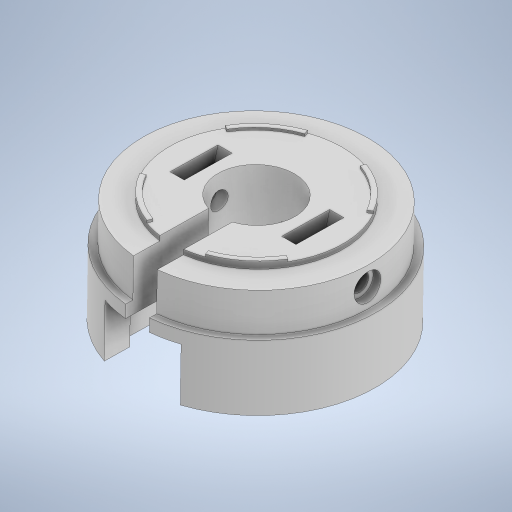
# Autodesk Inventor part: PiezoMount
Saved by Autodesk Inventor 2023 (Build 270158000, 158)
## iProperties
Created: 2023-02-27
Part Number: PiezoMount
Material: Generic
Document SubType Name: Modeling
Designer: maste
Density: 1 g/cm^3
Appearance: Default
Author: maste
Autodesk Inventor part; units mm, degrees
ref_plane "YZ Plane" through (0, 0, 0) normal (1, 0, 0) x (0, 1, 0)
ref_plane "XY Plane" through (0, 0, 0) normal (0, 0, 1) x (1, 0, 0)
sketch "Sketch1" plane through (0, 0, 0) normal (0, 0, 1) x (1, 0, 0)
  circle A0 centre (0, 0) radius 25
  dimension "d2" = 50
  constraints: 1 centre point, 1 coincident
  measures "d2" diameter of A0
extrude "piezo surface" add sketch "Sketch1" along normal blind 8
sketch "Sketch4" plane through (0, 0, 0) normal (0, 0, -1) x (-1, 0, 0)
  circle A0 centre (0, 0) radius 25 projected
extrude "Depth extension to surface" add sketch "Sketch4" along normal blind 3.62
sketch "Sketch2" plane through (0, 0, 8) normal (0, 0, 1) x (1, 0, 0)
  circle A0 centre (0, 0) radius 17.95
  circle A1 centre (0, 0) radius 18.75
  line L0 (0, 0) -> (18.75, 0)
  arc A2 (18.75, 0) -> (16.238, 9.375) centre (0, 0) ccw
  line L1 (0, 0) -> (16.238, 9.375) construction
  line L2 (0, 0) -> (18.75, 0) construction
  line L3 (16.238, 9.375) -> (15.5452, 8.975)
  line L4 (0, 0) -> (0, 18.75)
  line L5 (0, 0) -> (0, -18.75)
  line L6 (0, 0) -> (-18.75, 0)
  line L7 (0, 0) -> (-16.238, -9.375)
  line L8 (0, 0) -> (-9.375, 16.238)
  line L9 (0, 0) -> (9.375, -16.238)
  point P0 (17.95, 0)
  point P1 (8.975, -15.5452)
  point P2 (0, -17.95)
  point P3 (-15.5452, -8.975)
  point P4 (-17.95, 0)
  point P5 (-8.975, 15.5452)
  point P6 (0, 17.95)
  dimension "d3" = 35.9
  dimension "d4" = 37.5
  dimension "d5" = 30
  constraints: 20 end point, 4 point on line, 3 coincident, 2 perpendicular, 2 point on circle, 1 centre point, 1 horizontal, 1 vertical, 12 other
  measures "d5" angle of L2 L1
sketch "Sketch3" plane through (0, 0, 8) normal (0, 0, 1) x (1, 0, 0)
  line L0 (0, 0) -> (8.975, -15.5452)
  arc A0 (17.95, 0) -> (15.5452, 8.975) centre (0, 0) ccw projected
  line L1 (0, 0) -> (17.95, 0)
  arc A1 (0, -17.95) -> (8.975, -15.5452) centre (0, 0) ccw projected
  line L2 (8.975, -15.5452) -> (17.95, 0)
  line L3 (13.4625, -7.7726) -> (0, 0)
  line L4 (13.4625, -7.7726) -> (4.8022, -2.7726)
  line L5 (13.4625, -7.7726) -> (4.8022, -2.7726)
  line L6 (13.4625, -7.7726) -> (4.8022, -2.7726)
  line L7 (4.8022, -2.7726) -> (6.0522, -0.6075)
  line L8 (6.0522, -0.6075) -> (14.7125, -5.6075)
  line L9 (14.7125, -5.6075) -> (13.4625, -7.7726)
  line L10 (13.4625, -7.7726) -> (4.8022, -2.7726)
  line L11 (4.8022, -2.7726) -> (3.5522, -4.9376)
  line L12 (3.5522, -4.9376) -> (12.2125, -9.9376)
  line L13 (12.2125, -9.9376) -> (13.4625, -7.7726)
  line L14 (12.2125, -9.9376) -> (14.7125, -5.6075)
  line L15 (14.7125, -5.6075) -> (16.4446, -6.6075)
  line L16 (16.4446, -6.6075) -> (13.9446, -10.9376)
  line L17 (13.9446, -10.9376) -> (12.2125, -9.9376)
  line L18 (-4.802, 2.7724) -> (-3.552, 4.9375)
  line L19 (-3.552, 4.9375) -> (-13.9443, 10.9375)
  line L20 (-4.802, 2.7724) -> (-6.052, 0.6074)
  line L21 (-6.052, 0.6074) -> (-16.4443, 6.6074)
  line L22 (-16.4443, 6.6074) -> (-23.8055, 10.8574)
  line L23 (-23.8055, 10.8574) -> (-21.3055, 15.1875)
  line L24 (-21.3055, 15.1875) -> (-13.9443, 10.9375)
  line L25 (-5.5448, 2.5) -> (-17.5448, 2.5)
  line L26 (-5.5448, 0) -> (-5.5448, 2.5)
  line L27 (-5.5448, 0) -> (-5.5448, -2.5)
  line L28 (-5.5448, -2.5) -> (-17.5448, -2.5)
  line L29 (-17.5448, -2.5) -> (-26.0448, -2.5)
  line L30 (-26.0448, -2.5) -> (-26.0448, 2.5)
  line L31 (-26.0448, 2.5) -> (-17.5448, 2.5)
  point P0 (14.7125, -5.6075)
  point P1 (12.2125, -9.9376)
  point P2 (12.2125, -9.9376)
  dimension "d37" = 10
  dimension "d38" = 2.5
  dimension "d39" = 2.5
  dimension "d40" = 2
  dimension "d49" = 10
  dimension "d69" = 30
  dimension "d71" = 20.5
  dimension "d72" = 5
  constraints: 64 end point, 7 parallel, 4 collinear, 3 perpendicular, 1 midpoint, 1 point on line, 15 other
  measures "d37" distance of L3.start L4.end
  measures "d38" distance of L4.end L7.end
  measures "d39" distance of L11.end L4.end
  measures "d40" distance of L8.end L15.end
  measures "d49" distance between parallel lines of L11 L13
  measures "d71" distance between parallel lines of L30 L27
  measures "d72" distance between parallel lines of L25 L28
extrude "Microphone Wire Hole" cut sketch "Sketch3" against normal blind 14 contours L26 L27 L28 L29 L30 L31 L25 L21 L20 | L20 L21 L25 L26
sketch "Sketch5" plane through (0, 0, -3.62) normal (0, 0, -1) x (-1, 0, 0)
  line L0 (16, -16) -> (-16, -16)
  line L1 (-16, -16) -> (-16, 16)
  line L2 (-16, 16) -> (16, 16)
  line L3 (16, 16) -> (16, -16)
  line L4 (16, -16) -> (-16, 16) construction
  line L5 (-16, -16) -> (16, 16) construction
  circle A0 centre (0, 0) radius 20
  point P0 (-12, -16)
  point P1 (12, -16)
  point P2 (-16, 12)
  point P3 (-16, -12)
  point P4 (16, 12)
  point P5 (16, -12)
  point P6 (12, 16)
  point P7 (-12, 16)
  dimension "d18" = 32
  dimension "d19" = 32
  dimension "d54" = 40
  constraints: 12 end point, 2 midpoint, 2 parallel, 1 centre point, 1 coincident, 1 horizontal, 1 perpendicular
  measures "d18" distance of L0.start L0.end
  measures "d19" distance of L0.end L1.end
  measures "d54" diameter of A0
extrude "Circuit chamber" cut sketch "Sketch5" against normal blind 3
sketch "Sketch6" plane through (-16, -16, -3.62) normal (1, 0, 0) x (0, 0, -1)
  line L0 (0, 4) -> (0, 0) projected
  line L1 (0, 32) -> (-3, 32) projected
  line L2 (-3, 32) -> (-3, 28) projected
  line L3 (0, 0) -> (-3, 0) projected
  line L4 (-3, 4) -> (-3, 0) projected
  line L5 (0, 32) -> (0, 28) projected
  line L6 (0, 4) -> (-3, 4) projected
  line L7 (0, 18.5) -> (0, 13.5) projected
  line L8 (-11.62, 13.5) -> (-11.62, 18.5) projected
  line L9 (-3, 32) -> (-3, 28) projected
  line L10 (-3, 32) -> (-3, 32) projected
  line L11 (-3, 28) -> (-3, 32) projected
  line L12 (-3, 4) -> (-3, 28) projected
  line L13 (-3, 0) -> (-3, 4) projected
  line L14 (-3, 0) -> (-3, 0) projected
  line L15 (-3, 4) -> (-3, 0) projected
  line L16 (-3, 13.5) -> (-3, 4) projected
  line L17 (0, 18.5) -> (0, 13.5) projected
  line L18 (0, 13.5) -> (0, 4) projected
  line L19 (0, 4) -> (0, 0) projected
  line L20 (0, 0) -> (0, 0) projected
  line L21 (0, 0) -> (0, 4) projected
  line L22 (0, 4) -> (0, 28) projected
  line L23 (0, 28) -> (0, 32) projected
  line L24 (0, 32) -> (0, 32) projected
  line L25 (0, 32) -> (0, 28) projected
  line L26 (-11.62, 16) -> (0, 16)
  line L27 (0, 16) -> (-3, 16)
  line L28 (-3, 16) -> (-3, 24)
  line L29 (-3, 24) -> (0, 24)
  line L30 (0, 24) -> (0, 16)
  line L31 (0, 16) -> (-3, 16)
  line L32 (-3, 16) -> (-3, 8)
  line L33 (-3, 8) -> (0, 8)
  line L34 (0, 8) -> (0, 16)
  line L35 (0, 28) -> (0, 18.5) projected
  line L36 (-3, 18.5) -> (-3, 13.5) projected
  line L37 (-3, 28) -> (-3, 18.5) projected
  line L38 (0, 28) -> (-3, 28) projected
  line L39 (0, 18.5) -> (-11.62, 18.5) projected
  line L40 (-11.62, 13.5) -> (0, 13.5) projected
  point P0 (0, -9)
  point P1 (0, 41)
  point P2 (-11, 41)
  point P3 (-11, -9)
  point P4 (0, -9)
  point P5 (0, 41)
  point P6 (-3, 4)
  point P7 (-3, 8)
  point P8 (0, 8)
  point P9 (-3, 16)
  point P10 (-3, 13.5)
  point P11 (0, 13.5)
  point P12 (0, 18.5)
  dimension "d65" = 8
  dimension "d66" = 8
  constraints: 18 end point, 4 parallel, 2 horizontal, 2 midpoint, 2 perpendicular, 2 point on line
  measures "d65" distance of L27.end L28.end
  measures "d66" distance of L32.end L31.end
extrude "port vent" cut sketch "Sketch6" against normal blind 30 contours L33 L12 L40 L18 | L39 L12 L29 L22
sketch "Sketch7" plane through (0, 0, -3.62) normal (0, 0, -1) x (-1, 0, 0)
  line L0 (0, 0) -> (0, -17.5)
  line L1 (0, 0) -> (0, 17.5)
  dimension "d25" = 17.5
  dimension "d26" = 17.5
  constraints: 4 end point, 2 coincident, 2 vertical
  measures "d25" distance of L0.start L0.end
  measures "d26" distance of L0.start L1.end
hole "screw holes" at (0, 17.5, -3.62) at (0, -17.5, -3.62) direction (0, 0, 1) diameter 3.7 depth 4 tip angle 118
sketch "Sketch8" plane through (0, 0, -3.62) normal (0, 0, -1) x (-1, 0, 0)
  circle A0 centre (0, 0) radius 22.75
  line L0 (21.4137, 11) -> (22.4499, 11) projected
  line L1 (22.4499, 11) -> (19.9139, 11)
  arc A1 (23.6854, 8) -> (23.6854, -8) centre (0, 0) ccw projected
  line L2 (24.6779, -4) -> (22.3956, -4)
  arc A2 (24.8747, 2.5) -> (24.8747, -2.5) centre (0, 0) ccw projected
  arc A3 (-16, 12) -> (-16, -12) centre (0, 0) ccw projected
  arc A4 (-12, -16) -> (12, -16) centre (0, 0) ccw projected
  point P0 (12.5, 7.5)
  point P1 (15.0629, 9)
  point P2 (19.2094, 16)
  point P3 (19.2094, -16)
  point P4 (19.9139, 11)
  point P5 (16.7033, 11)
  point P6 (24.6779, 4)
  point P7 (21.9317, -12)
  dimension "d34" = 45.5
  constraints: 4 end point, 2 point on circle, 1 centre point, 1 coincident, 1 horizontal, 1 parallel, 1 other
  measures "d34" diameter of A0
sketch "Sketch10" plane through (0, 0, -3.62) normal (0, 0, -1) x (-1, 0, 0)
  arc A0 (23.6854, 8) -> (23.6854, -8) centre (0, 0) ccw projected
  arc A1 (16, -12) -> (18.3303, -8) centre (0, 0) ccw projected
  line L0 (16, -16) -> (12, -16) projected
  arc A2 (-12, -16) -> (12, -16) centre (0, 0) ccw projected
  line L1 (-12, -16) -> (-16, -16) projected
  line L2 (-16, -16) -> (-16, -12) projected
  arc A3 (-16, 12) -> (-16, -12) centre (0, 0) ccw projected
  line L3 (-16, 12) -> (-16, 16) projected
  line L4 (-16, 16) -> (-12, 16) projected
  arc A4 (12, 16) -> (-12, 16) centre (0, 0) ccw projected
  line L5 (12, 16) -> (16, 16) projected
  line L6 (16, 16) -> (16, 12) projected
  line L7 (18.3303, 8) -> (23.6854, 8) projected
  line L8 (23.6854, -8) -> (18.3303, -8) projected
  line L9 (16, -12) -> (16, -16) projected
  arc A5 (18.3303, 8) -> (16, 12) centre (0, 0) ccw projected
extrude "Base Extension" add sketch "Sketch10" along normal blind 10
sketch "Sketch13" plane through (0, 0, 8) normal (0, 0, 1) x (0, 1, 0)
  circle A0 centre (0, 0) radius 25
  circle A1 centre (0, 0) radius 23.5
  dimension "d55" = 47
  dimension "d59" = 50
  constraints: 2 centre point, 2 coincident
  measures "d55" diameter of A1
  measures "d59" diameter of A0
extrude "Rim for flush with diaphragm lock" cut sketch "Sketch13" against normal blind 8
sketch "Sketch14" plane through (-16, 12.1244, -3) normal (1, 0, 0) x (0, 0, -1)
  line L0 (10.62, -4.1244) -> (10.62, -20.1244) projected
  line L1 (-3, 11.3756) -> (-11, 11.3756) projected
  line L2 (-11, 11.3756) -> (-11, -35.6244) projected
  line L3 (-3, -9.6244) -> (-3, -14.6244) projected
  line L4 (-2.38, -20.1244) -> (10.62, -20.1244) projected
  line L5 (10.62, -4.1244) -> (-2.38, -4.1244) projected
  line L6 (-3, -14.6244) -> (-2.38, -14.6244) projected
  line L7 (-2.38, -14.6244) -> (-2.38, -20.1244) projected
  line L8 (-2.38, -4.1244) -> (-2.38, -9.6244) projected
  line L9 (-2.38, -9.6244) -> (-3, -9.6244) projected
  point P0 (-3, -12.1244)
  point P1 (-4, -2.6061)
  point P2 (-4, 1.724)
  point P3 (-11, -35.6244)
  constraints: 1 other
sketch "Sketch16" plane through (0, 0, 8) normal (0, 0, 1) x (1, 0, 0)
  circle A0 centre (0, 0) radius 18
  arc A1 (-23.3666, -2.5) -> (-23.3666, 2.5) centre (0, 0) ccw projected
  line L0 (-23.3666, 2.5) -> (-5.5448, 2.5) projected
  line L1 (-5.5448, 2.5) -> (-5.5448, -2.5) projected
  line L2 (-5.5448, -2.5) -> (-23.3666, -2.5) projected
  point P0 (-17.8255, -2.5)
  point P1 (-17.8255, 2.5)
  dimension "d73" = 36
  constraints: 1 centre point, 1 coincident
  measures "d73" diameter of A0
extrude "Extrusion11" add sketch "Sketch16" along normal blind 1 contours A0 L2 L1 L0 picked at (2.3035, 0)
sketch "Sketch17" plane through (0, 0, -13.62) normal (0, 0, -1) x (-1, 0, 0)
  arc A0 (12, 16) -> (-12, 16) centre (0, 0) ccw projected
  line L0 (12, 16) -> (-12, 16)
  line L1 (-12, 20.5) -> (12, 20.5)
  line L2 (12, 20.5) -> (12, 11.5)
  line L3 (12, 11.5) -> (-12, 11.5)
  line L4 (-12, 11.5) -> (-12, 20.5)
  line L5 (-12, 20.5) -> (12, 11.5) construction
  line L6 (12, 20.5) -> (-12, 11.5) construction
  arc A1 (-16, 12) -> (-16, -12) centre (0, 0) ccw projected
  line L7 (0, 0) -> (-20, 0)
  line L8 (-12, -20.5) -> (12, -20.5)
  line L9 (12, -20.5) -> (12, -11.5)
  line L10 (12, -11.5) -> (-12, -11.5)
  line L11 (-12, -11.5) -> (-12, -20.5)
  point P0 (0, 16)
  dimension "d76" = 9
  constraints: 24 end point, 4 symmetric about line, 3 midpoint, 2 parallel, 1 horizontal, 1 perpendicular, 1 point on circle
  measures "d76" distance of L1.end L2.end
extrude "Extrusion12" add sketch "Sketch17" against normal blind 4
fillet "Fillet1" radius 5 4 edges at (-12, -11.5, -11.62) (12, -11.5, -11.62) (12, 11.5, -11.62) (-12, 11.5, -11.62)
sketch "Sketch18" plane through (0, 0, -13.62) normal (0, 0, -1) x (-1, 0, 0)
  circle A0 centre (0, -17.5) radius 1.85 projected
  circle A1 centre (0, 17.5) radius 1.85 projected
  arc A2 (23.6854, 8) -> (23.6854, -8) centre (0, 0) ccw projected
  dimension "d87" = 17.5
  dimension "d88" = 17.5
  dimension "d92" = 3.7
  measures "d87" distance of A2.centre A1.centre
  measures "d88" distance of point (0, 0) A0.centre
  measures "d92" diameter of A0
extrude "Extrusion13" cut sketch "Sketch18" against normal blind 4
sketch "Sketch19" plane through (0, 0, -9.62) normal (0, 0, 1) x (1, 0, 0)
  circle A0 centre (0, 17.5) radius 1.85 projected
  arc A1 (-12, 16) -> (-7.0251, 11.5) centre (-7.0251, 16.5) ccw projected
  line L0 (-7.0251, 11.5) -> (7.0251, 11.5) projected
  arc A2 (7.0251, 11.5) -> (12, 16) centre (7.0251, 16.5) ccw projected
  arc A3 (12, 16) -> (-12, 16) centre (0, 0) ccw projected
  line L1 (-1.2512, 20.6061) -> (2.0643, 20.1366)
  circle A4 centre (0, -17.5) radius 1.85 projected
  arc A5 (12, -16) -> (7.0251, -11.5) centre (7.0251, -16.5) ccw projected
  line L2 (7.0251, -11.5) -> (-7.0251, -11.5) projected
  arc A6 (-7.0251, -11.5) -> (-12, -16) centre (-7.0251, -16.5) ccw projected
  arc A7 (-12, -16) -> (12, -16) centre (0, 0) ccw projected
  circle A8 centre (0, -17.5) radius 1.85 projected
  line L3 (3.5161, -17.7003) -> (1.5846, -20.6452)
  line L4 (1.5846, -20.6452) -> (-1.9315, -20.4449)
  line L5 (-1.9315, -20.4449) -> (-3.5161, -17.2997)
  line L6 (-3.5161, -17.2997) -> (-1.5846, -14.3548)
  line L7 (-1.5846, -14.3548) -> (1.9315, -14.5551)
  line L8 (1.9315, -14.5551) -> (3.5161, -17.7003)
  line L9 (1.7609, 20.55) -> (3.5218, 17.5)
  line L10 (3.5218, 17.5) -> (1.7609, 14.45)
  line L11 (1.7609, 14.45) -> (-1.7609, 14.45)
  line L12 (-1.7609, 14.45) -> (-3.5218, 17.5)
  line L13 (-3.5218, 17.5) -> (-1.7609, 20.55)
  line L14 (-1.7609, 20.55) -> (1.7609, 20.55)
  point P0 (-2.2178, -19.8766)
  point P1 (2.0788, -19.8917)
  dimension "d83" = 6.1
  dimension "d86" = 6.1
  constraints: 26 end point, 3 coincident, 28 other
  measures "d83" distance between parallel lines of L6 L3
  measures "d86" distance between parallel lines of L12 L9
extrude "Extrusion14" cut sketch "Sketch19" against normal blind 1 contours A0 | L13 L14 L1 L9 A3 | A3 L9 L10 L11 L12 L13 | L1 L14 L9 | L3 L4 L5 A7 | A7 L5 L6 L7 L8 L3
sketch "Sketch20" plane through (0, 0, -0.62) normal (0, 0, -1) x (-1, 0, 0)
  circle A0 centre (0, 17.5) radius 1.85 projected
  line L0 (-1.7609, 14.45) -> (1.7609, 14.45) projected
  line L1 (-3.5218, 17.5) -> (-1.7609, 14.45) projected
  line L2 (-1.7609, 20.55) -> (-3.5218, 17.5) projected
  line L3 (1.7609, 20.55) -> (-1.7609, 20.55) projected
  line L4 (3.5218, 17.5) -> (1.7609, 20.55) projected
  line L5 (1.7609, 14.45) -> (3.5218, 17.5) projected
  line L6 (1.5846, -14.3548) -> (-1.9315, -14.5551) projected
  line L7 (3.5161, -17.2997) -> (1.5846, -14.3548) projected
  line L8 (1.9315, -20.4449) -> (3.5161, -17.2997) projected
  line L9 (-3.5161, -17.7003) -> (-1.5846, -20.6452) projected
  line L10 (-1.9315, -14.5551) -> (-3.5161, -17.7003) projected
  circle A1 centre (0, -17.5) radius 1.85 projected
  line L11 (-1.5846, -20.6452) -> (1.9315, -20.4449) projected
  point P0 (0, 0)
  dimension "d91" = 6.1
  measures "d91" distance between parallel lines of L9 L7
extrude "Extrusion15" cut sketch "Sketch20" along normal blind 11 contours L1 L2 L3 L4 L5 L0 | L7 L8 L11 L9 L10 L6 | A1
sketch "Sketch21" plane through (0, 0, 0) normal (0, 1, 0) x (-1, 0, 0)
  line L0 (23.3666, 8) -> (23.3666, 0) projected
  line L1 (23.3666, 8) -> (23.3666, 8) projected
  line L2 (23.3666, 0) -> (23.3666, 8) projected
  line L3 (23.3666, 0) -> (23.3666, 0) projected
  line L4 (23.3666, 8) -> (23.3666, 0) projected
  line L5 (23.3666, 8) -> (23.3666, 8) projected
  line L6 (23.3666, 0) -> (23.3666, 8) projected
  line L7 (23.3666, 0) -> (23.3666, 0) projected
  line L8 (23.3666, 8) -> (23.3666, 0) projected
  line L9 (23.3666, 8) -> (23.3666, 8) projected
  line L10 (23.3666, 0) -> (23.3666, 8) projected
  line L11 (23.3666, 0) -> (23.3666, 0) projected
  line L12 (-23.5, 0) -> (-23.5, 8) projected
  line L13 (-23.5, 8) -> (-23.5, 0)
  line L14 (-23.5, 0) -> (-23.5, 8) projected
  line L15 (-23.5, 4) -> (23.3666, 4)
  line L16 (23.3666, 8) -> (23.3666, 0)
  line L17 (23.3666, 0) -> (-23.5, 8)
  line L18 (-23.5, 0) -> (23.3666, 8)
  point P0 (-0.0667, 4)
  constraints: 10 end point, 3 midpoint, 2 collinear
ref_plane "Work Plane2" through (-23.3666, -27.5, -0.62) normal (0, -1, 0) x (1, 0, 0)
hole "Hole2" at (0.0667, 0, 4) direction (0, -1, 0) diameter 3.7 end through all
hole "Hole3" at (0.0667, 0, 4) direction (0, 1, 0) diameter 3.7 end through all
sketch "Sketch23" plane through (-23.3666, -27.5, -0.62) normal (0, -1, 0) x (1, 0, 0)
  spline S0 degree 7 poles (23.4333, 6.47) (23.3306, 6.47) (23.228, 6.4633) (23.1263, 6.4501) (23.0264, 6.4303) (22.9289, 6.4045) (22.8347, 6.3732) (22.557, 6.2617) (22.3866, 6.1657) (22.2343, 6.0531) (22.1005, 5.9277) (21.9851, 5.7925) (21.8878, 5.6504) (21.743, 5.384) (21.6893, 5.2608) (21.6467, 5.1351) (21.615, 5.0075) (21.5939, 4.8787) (21.5833, 4.7494) (21.5833, 4.4432) (21.603, 4.2664) (21.6424, 4.0912) (21.7019, 3.9189) (21.782, 3.7513) (21.8837, 3.5908) (22.1047, 3.3238) (22.2157, 3.2123) (22.3412, 3.1089) (22.4807, 3.0162) (22.6334, 2.9367) (22.7981, 2.8731) (23.1313, 2.7875) (23.2967, 2.7624) (23.4659, 2.7549) (23.6352, 2.7657) (23.8006, 2.7944) (23.9587, 2.8391) (24.3421, 2.9889) (24.5511, 3.1138) (24.7312, 3.2629) (24.8825, 3.4294) (25.0055, 3.6081) (25.1013, 3.7945) (25.2493, 4.1996) (25.2951, 4.4205) (25.3097, 4.6444) (25.2936, 4.8686) (25.2465, 5.0902) (25.1673, 5.306) (24.9375, 5.724) (24.7801, 5.9332) (24.5794, 6.1251) (24.3373, 6.2866) (24.0591, 6.4053) (23.7535, 6.47) (23.4333, 6.47) knots 0 0 0 0 0 0 0 0 0.052516 0.052516 0.052516 0.052516 0.052516 0.052516 0.161373 0.161373 0.161373 0.161373 0.161373 0.161373 0.250167 0.250167 0.250167 0.250167 0.250167 0.250167 0.371544 0.371544 0.371544 0.371544 0.371544 0.371544 0.466188 0.466188 0.466188 0.466188 0.466188 0.466188 0.551622 0.551622 0.551622 0.551622 0.551622 0.551622 0.688001 0.688001 0.688001 0.688001 0.688001 0.688001 0.841193 0.841193 0.841193 0.841193 0.841193 0.841193 1 1 1 1 1 1 1 1 projected
  arc A0 (23.4333, 6.47) -> (23.4333, 2.77) centre (23.4333, 4.62) ccw
  circle A1 centre (23.4333, 4.62) radius 2.825
  dimension "d163" = 5.65
  constraints: 2 centre point, 2 point on circle, 1 coincident, 5 other
  measures "d163" diameter of A1
extrude "Extrusion16" cut sketch "Sketch23" against normal blind 5.75
ref_plane "Work Plane3" through (0, 23.5, 0) normal (0, 1, 0) x (-1, 0, 0)
sketch "Sketch24" plane through (0, 23.5, 0) normal (0, 1, 0) x (-1, 0, 0)
  spline S0 degree 7 poles (-0.0667, 5.85) (0.036, 5.85) (0.1386, 5.8433) (0.2403, 5.8301) (0.3403, 5.8103) (0.4377, 5.7845) (0.5319, 5.7532) (0.8097, 5.6417) (0.9801, 5.5457) (1.1324, 5.4331) (1.2662, 5.3077) (1.3815, 5.1725) (1.4788, 5.0304) (1.6237, 4.764) (1.6773, 4.6408) (1.7199, 4.5151) (1.7517, 4.3875) (1.7728, 4.2587) (1.7833, 4.1294) (1.7833, 3.8232) (1.7636, 3.6464) (1.7242, 3.4712) (1.6648, 3.2989) (1.5846, 3.1313) (1.4829, 2.9708) (1.262, 2.7038) (1.1509, 2.5923) (1.0254, 2.4889) (0.886, 2.3962) (0.7333, 2.3167) (0.5685, 2.2531) (0.2353, 2.1675) (0.07, 2.1424) (-0.0993, 2.1349) (-0.2685, 2.1457) (-0.434, 2.1744) (-0.592, 2.2191) (-0.9755, 2.3689) (-1.1844, 2.4938) (-1.3646, 2.6429) (-1.5159, 2.8094) (-1.6389, 2.9881) (-1.7347, 3.1745) (-1.8827, 3.5796) (-1.9284, 3.8005) (-1.943, 4.0244) (-1.9269, 4.2486) (-1.8799, 4.4702) (-1.8007, 4.686) (-1.5709, 5.104) (-1.4134, 5.3132) (-1.2128, 5.5051) (-0.9706, 5.6666) (-0.6925, 5.7853) (-0.3869, 5.85) (-0.0667, 5.85) knots 0 0 0 0 0 0 0 0 0.052516 0.052516 0.052516 0.052516 0.052516 0.052516 0.161373 0.161373 0.161373 0.161373 0.161373 0.161373 0.250167 0.250167 0.250167 0.250167 0.250167 0.250167 0.371544 0.371544 0.371544 0.371544 0.371544 0.371544 0.466188 0.466188 0.466188 0.466188 0.466188 0.466188 0.551622 0.551622 0.551622 0.551622 0.551622 0.551622 0.688001 0.688001 0.688001 0.688001 0.688001 0.688001 0.841193 0.841193 0.841193 0.841193 0.841193 0.841193 1 1 1 1 1 1 1 1 projected
  arc A0 (-1.9167, 4) -> (-1.9167, 4) centre (-0.0668, 4) ccw
  circle A1 centre (-0.0668, 4) radius 2.825
  dimension "d164" = 5.65
  constraints: 2 centre point, 2 coincident, 2 point on circle, 2 other
  measures "d164" diameter of A1
extrude "Extrusion17" cut sketch "Sketch24" against normal blind 1.75
sketch "Sketch26" plane through (0, 0, 9) normal (0, 0, 1) x (1, 0, 0)
  line L0 (-1.7589, -21.75) -> (1.9411, -21.75) projected
  line L1 (1.9411, 21.75) -> (-1.7589, 21.75) projected
  line L2 (-2.7339, 21.75) -> (2.9161, 21.75) projected
  line L3 (0.0911, 21.75) -> (0.0911, -21.75)
  line L4 (0.0911, 21.75) -> (0.0911, 11.75)
  line L5 (0.0911, -21.75) -> (0.0911, -11.75)
  line L6 (3.1411, -13.25) -> (-2.9589, -13.25)
  line L7 (-2.9589, -13.25) -> (-2.9589, -10.25)
  line L8 (-2.9589, -10.25) -> (3.1411, -10.25)
  line L9 (3.1411, -10.25) -> (3.1411, -13.25)
  line L10 (3.1411, -13.25) -> (-2.9589, -10.25) construction
  line L11 (-2.9589, -13.25) -> (3.1411, -10.25) construction
  line L12 (3.1411, 10.25) -> (-2.9589, 10.25)
  line L13 (-2.9589, 10.25) -> (-2.9589, 13.25)
  line L14 (-2.9589, 13.25) -> (3.1411, 13.25)
  line L15 (3.1411, 13.25) -> (3.1411, 10.25)
  line L16 (3.1411, 10.25) -> (-2.9589, 13.25) construction
  line L17 (-2.9589, 10.25) -> (3.1411, 13.25) construction
  point P0 (0, 0)
  dimension "d124" = 10
  dimension "d125" = 10
  dimension "d126" = 6.1
  dimension "d127" = 3
  dimension "d128" = 6.1
  dimension "d129" = 3
  constraints: 30 end point, 6 midpoint, 4 parallel, 4 perpendicular, 2 point on line
  measures "d124" distance of L3.start L4.end
  measures "d125" distance of L3.end L5.end
  measures "d126" distance of L6.start L6.end
  measures "d127" distance of L6.end L7.end
  measures "d128" distance of L12.start L12.end
  measures "d129" distance of L12.end L13.end
extrude "Extrusion19" cut sketch "Sketch26" against normal blind 9
sketch "Sketch27" plane through (0, 0, -0.62) normal (0, 0, -1) x (-1, 0, 0)
  circle A0 centre (0, 17.5) radius 1.85 projected
  circle A1 centre (0, -17.5) radius 1.85 projected
  arc A2 (7.0251, 11.5) -> (12, 16) centre (7.0251, 16.5) ccw projected
  line L0 (12, 16) -> (16, 16) projected
  line L1 (16, 16) -> (16, 12) projected
  arc A3 (18.3303, 8) -> (16, 12) centre (0, 0) ccw projected
  line L2 (18.3303, 8) -> (23.6854, 8) projected
  arc A4 (23.6854, 8) -> (23.6854, -8) centre (0, 0) ccw projected
  line L3 (23.6854, -8) -> (18.3303, -8) projected
  arc A5 (16, -12) -> (18.3303, -8) centre (0, 0) ccw projected
  line L4 (16, -12) -> (16, -16) projected
  line L5 (16, -16) -> (12, -16) projected
  arc A6 (12, -16) -> (7.0251, -11.5) centre (7.0251, -16.5) ccw projected
  line L6 (7.0251, -11.5) -> (-7.0251, -11.5) projected
  arc A7 (-7.0251, -11.5) -> (-12, -16) centre (-7.0251, -16.5) ccw projected
  line L7 (-12, -16) -> (-16, -16) projected
  line L8 (-16, -16) -> (-16, -12) projected
  arc A8 (-16, 12) -> (-16, -12) centre (0, 0) ccw projected
  line L9 (-16, 12) -> (-16, 16) projected
  line L10 (-16, 16) -> (-12, 16) projected
  arc A9 (-12, 16) -> (-7.0251, 11.5) centre (-7.0251, 16.5) ccw projected
  line L11 (-7.0251, 11.5) -> (7.0251, 11.5) projected
  line L12 (18.3303, 8) -> (-5.6697, 8)
  line L13 (-5.6697, 8) -> (-5.6697, -8)
  line L14 (-5.6697, -8) -> (18.3303, -8)
  line L15 (18.3303, -8) -> (18.3303, 8)
  line L16 (-5.6697, 0) -> (18.3303, 0)
  line L17 (18.3303, 0) -> (18.3303, 10)
  line L18 (18.3303, 10) -> (-5.6697, 10)
  line L19 (-5.6697, 10) -> (-5.6697, 0)
  line L20 (-5.6697, 0) -> (18.3303, 0)
  line L21 (18.3303, 0) -> (18.3303, -10)
  line L22 (18.3303, -10) -> (-5.6697, -10)
  line L23 (-5.6697, -10) -> (-5.6697, 0)
  line L24 (20.3303, -11.5) -> (20.3303, 11.5)
  line L25 (20.3303, 11.5) -> (-7.6697, 11.5)
  line L26 (-7.6697, 11.5) -> (-7.6697, -11.5)
  line L27 (-7.6697, -11.5) -> (20.3303, -11.5)
  line L28 (20.3303, -11.5) -> (-7.6697, 11.5) construction
  line L29 (20.3303, 11.5) -> (-7.6697, -11.5) construction
  point P0 (6.3303, 0)
  point P1 (-7.0251, -11.5)
  point P2 (16.3631, -11.5)
  point P3 (17.3205, -10)
  point P4 (-5.6697, -8)
  point P5 (17.3205, 10)
  point P6 (16.3631, 11.5)
  dimension "d132" = 24
  dimension "d133" = 16
  dimension "d134" = 10
  dimension "d135" = 10
  dimension "d136" = 28
  constraints: 36 end point, 8 parallel, 4 midpoint, 4 perpendicular, 3 horizontal, 1 point on line, 1 vertical
  measures "d132" distance of L14.end L13.end
  measures "d133" distance of L14.end L2.start
  measures "d134" distance of L17.end L16.end
  measures "d135" distance of L20.end L21.end
  measures "d136" distance of L25.end L24.end
extrude "Extrusion20" add sketch "Sketch27" along normal blind 5 contours L25 A3 L18 L19 L13 L23 L22 A5 L27 L6 L26 L11
sketch "Sketch28" plane through (0, 0, -13.62) normal (0, 0, -1) x (-1, 0, 0)
  point P0 (0, 0)
chamfer "Chamfer1" distance 2 distance2 8 1 edges at (3.1411, -11.75, 9) measured on face at (3.6411, -11.75, 9)
chamfer "Chamfer2" distance 2 distance2 8 1 edges at (-2.9589, -11.75, 9) measured on face at (-3.4589, -11.75, 9)
chamfer "Chamfer3" distance 2 distance2 8 1 edges at (3.1411, 11.75, 9) measured on face at (3.6411, 11.75, 9)
chamfer "Chamfer4" distance 2 distance2 8 1 edges at (-2.9589, 11.75, 9) measured on face at (-3.4589, 11.75, 9)
sketch "Sketch30" plane through (0, 0, -0.62) normal (0, 0, -1) x (-1, 0, 0)
  line L0 (17.3205, 10) -> (-5.6697, 10) projected
  line L1 (-5.6697, 10) -> (-5.6697, -10) projected
  line L2 (-5.6697, -10) -> (17.3205, -10) projected
  arc A0 (17.3205, -10) -> (18.3303, -8) centre (0, 0) ccw projected
  line L3 (18.3303, -8) -> (23.6854, -8) projected
  line L4 (5.5448, -2.5) -> (24.8747, -2.5) projected
  line L5 (5.5448, 2.5) -> (5.5448, -2.5) projected
  line L6 (24.8747, 2.5) -> (5.5448, 2.5) projected
  line L7 (18.3303, 8) -> (23.6854, 8) projected
  arc A1 (18.3303, 8) -> (17.3205, 10) centre (0, 0) ccw projected
  arc A2 (23.6854, -8) -> (24.8747, -2.5) centre (0, 0) ccw projected
  arc A3 (24.8747, 2.5) -> (23.6854, 8) centre (0, 0) ccw projected
extrude "Extrusion21" add sketch "Sketch30" along normal blind 2
sketch "Sketch31" plane through (0, 0, 9) normal (0, 0, 1) x (1, 0, 0)
  circle A0 centre (0, 0) radius 8
  dimension "d153" = 16
  constraints: 1 centre point, 1 coincident
  measures "d153" diameter of A0
extrude "Extrusion22" cut sketch "Sketch31" against normal blind 15
sketch "Sketch32" plane through (0, 0, 9) normal (0, 0, 1) x (1, 0, 0)
  arc A0 (-17.8255, -2.5) -> (-17.8255, 2.5) centre (0, 0) ccw projected
  circle A1 centre (0, 0) radius 18
  arc A2 (18, 0) -> (0, 18) centre (0, 0) ccw
  arc A3 (-16.8352, -2.3611) -> (-16.8352, 2.3611) centre (0, 0) ccw
  line L0 (0, 0) -> (18, 0) construction
  line L1 (0, 0) -> (18, 0) construction
  line L2 (0, 0) -> (-16.9145, 6.1564)
  line L3 (0, 0) -> (18, 0) construction
  line L4 (0, 0) -> (-9, 15.5885)
  line L5 (0, 0) -> (18, 0) construction
  line L6 (-9, 15.5885) -> (9, -15.5885)
  line L7 (-16.9145, 6.1564) -> (16.9145, -6.1564)
  line L8 (0, 0) -> (-16.9145, -6.1564)
  line L9 (0, 0) -> (-9, -15.5885)
  line L10 (-9, -15.5885) -> (9, 15.5885)
  line L11 (-16.9145, -6.1564) -> (16.9145, 6.1564)
  point P0 (-8.5, -14.7224)
  point P1 (-15.9748, -5.8143)
  point P2 (16.9145, -6.1564)
  point P3 (15.9748, -5.8143)
  point P4 (8.5, -14.7224)
  point P5 (15.9748, 5.8143)
  point P6 (9, 15.5885)
  point P7 (8.5, 14.7224)
  point P8 (-8.5, 14.7224)
  point P9 (-15.9748, 5.8143)
  dimension "d156" = 1
  dimension "d159" = 160
  dimension "d160" = 120
  constraints: 24 end point, 9 point on circle, 4 horizontal, 2 centre point, 2 equal length, 1 coincident, 10 other
  measures "d156" radial gap between concentric circles of A0 A3
  measures "d159" angle of L3 L2
  measures "d160" angle of L5 L4
extrude "Extrusion23" add sketch "Sketch32" along normal blind 0.5 contours L8 A3 L9 A0 | A0 L4 A3 L2 | L6 A3 L7 A0 | L10 A0 L11 A3
sketch "Sketch35" plane through (0, 0, -13.62) normal (0, 0, -1) x (-1, 0, 0)
  arc A0 (-5.6697, 5.644) -> (-7.6697, 2.275) centre (0, 0) ccw projected
  line L0 (-5.6697, 5.644) -> (-5.6697, 10) projected
  line L1 (-5.6697, 10) -> (17.3205, 10) projected
  arc A1 (17.3205, 10) -> (16.3631, 11.5) centre (0, 0) ccw projected
  line L2 (16.3631, 11.5) -> (-7.6697, 11.5) projected
  line L3 (-7.6697, 11.5) -> (-7.6697, 2.275) projected
  arc A2 (-7.6697, -2.275) -> (-5.6697, -5.644) centre (0, 0) ccw projected
  line L4 (-7.6697, -2.275) -> (-7.6697, -11.5) projected
  line L5 (-7.6697, -11.5) -> (16.3631, -11.5) projected
  arc A3 (16.3631, -11.5) -> (17.3205, -10) centre (0, 0) ccw projected
  line L6 (17.3205, -10) -> (-5.6697, -10) projected
  line L7 (-5.6697, -10) -> (-5.6697, -5.644) projected
  line L8 (17.3205, 10) -> (5.1275, 10)
  line L9 (5.1275, 10) -> (5.1275, 16.3135)
  line L10 (5.1275, 16.3135) -> (17.3205, 16.3135)
  line L11 (17.3205, 16.3135) -> (17.3205, 10)
  line L12 (17.3205, -10) -> (-5.6697, -10) projected
  arc A4 (17.8255, 2.5) -> (17.8255, -2.5) centre (0, 0) ccw projected
  line L13 (17.3205, -10) -> (6.3107, -10)
  line L14 (6.3107, -10) -> (6.3107, -16.8575)
  line L15 (6.3107, -16.8575) -> (17.3205, -16.8575)
  line L16 (17.3205, -16.8575) -> (17.3205, -10)
  point P0 (6.3107, -11.5)
  point P1 (5.1275, 11.5)
  constraints: 16 end point, 4 parallel, 2 horizontal, 2 perpendicular, 1 point on circle
extrude "Extrusion24" add sketch "Sketch35" against normal blind 4
body "Solid1"
